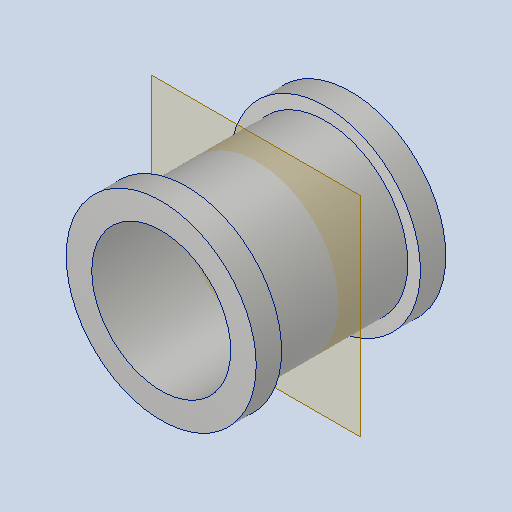
# Autodesk Inventor part: EL2-007
Saved by Autodesk Inventor 2023.4 (Build 274418000, 418)
## iProperties
Created: 2025-01-11
Part Number: EL2-007
Material: Aluminum 6061
Document SubType Name: Modeling
Designer: mavericks
Density: 2.7 g/cm^3
Appearance: Aluminum - Flat
Author: mavericks
Autodesk Inventor part; units mm, degrees
ref_plane "YZ Plane" through (0, 0, 0) normal (1, 0, 0) x (0, 1, 0)
ref_plane "XZ Plane" through (0, 0, 0) normal (0, 1, 0) x (-1, 0, 0)
sketch "Sketch1" plane through (0, 0, 0) normal (0, 0, 1) x (1, 0, 0)
  line L0 (-12.7, 76.2) -> (12.7, 76.2) construction
  line L1 (12.7, 76.2) -> (12.7, -76.2) construction
  line L2 (12.7, -76.2) -> (-12.7, -76.2) construction
  line L3 (-12.7, -76.2) -> (-12.7, 76.2) construction
  line L4 (-12.7, 76.2) -> (12.7, -76.2) construction
  line L5 (12.7, 76.2) -> (-12.7, -76.2) construction
  line L6 (19.05, 76.2) -> (44.45, 76.2) construction
  line L7 (44.45, 76.2) -> (44.45, -76.2) construction
  line L8 (44.45, -76.2) -> (19.05, -76.2) construction
  line L9 (19.05, -76.2) -> (19.05, 76.2) construction
  line L10 (19.05, 76.2) -> (44.45, -76.2) construction
  line L11 (44.45, 76.2) -> (19.05, -76.2) construction
  circle A0 centre (2.7686, 0) radius 8.6995
  line L12 (11.1125, -57.0186) -> (11.1125, 57.0186) construction
  line L13 (11.1125, 57.0186) -> (-14.2875, -95.3814) construction
  line L14 (-14.2875, -95.3814) -> (-14.2875, 95.3814) construction
  line L15 (-14.2875, 95.3814) -> (11.1125, -57.0186) construction
  line L16 (13.081, 27.2802) -> (13.081, -0.0011) construction
  circle A1 centre (2.7686, 0) radius 10.3124
  point P0 (0, 0)
  point P1 (31.75, 0)
  point P2 (0, 0)
  point P3 (0, 76.2)
  point P4 (31.75, 76.2)
  point P5 (0, 0)
  dimension "d1" = 25.4
  dimension "d2" = 152.4
  dimension "d3" = 25.4
  dimension "d4" = 152.4
  dimension "d5" = 6.35
  dimension "d6" = 17.399
  dimension "d7" = 1.5875
  dimension "d8" = 0.381
  dimension "d11" = 20.6248
  dimension "d21" = 9.9314
  constraints: 34 end point, 6 midpoint, 5 parallel, 2 centre point, 2 coincident, 2 horizontal, 2 horizontal alignment, 2 perpendicular, 1 tangent, 1 vertical, 3 other
  measures "d1" distance of L1.end L2.end
  measures "d2" distance of L0.end L1.end
  measures "d3" distance of L7.end L8.end
  measures "d4" distance of L6.end L7.end
  measures "d5" distance between parallel lines of L9 L1
  measures "d6" diameter of A0
  measures "d7" distance between parallel lines of L1 L12
  measures "d8" distance between parallel lines of L1 L16
  measures "d11" diameter of A1
  measures "d21" distance from line of A0.centre L1
extrude "Extrusion1" add sketch "Sketch1" along normal mid plane 17.399
sketch "Sketch2" plane through (2.7686, 0, 8.6995) normal (0, 0, 1) x (1, 0, 0)
  circle A0 centre (0, 0) radius 10.3124 projected
  circle A1 centre (0, 0) radius 11.8999
  circle A2 centre (0, 0) radius 8.6995 projected
  point P0 (-2.7686, 0)
  dimension "d14" = 1.5875
  constraints: 1 centre point
  measures "d14" radial gap between concentric circles of A0 A1
extrude "Extrusion2" add sketch "Sketch2" along normal blind 3.175 contours A0 | A1
sketch "Sketch3" plane through (2.7686, 0, -8.6995) normal (0, 0, -1) x (-1, 0, 0)
  circle A0 centre (0, 0) radius 10.3124 projected
  circle A1 centre (0, 0) radius 11.8999
  circle A2 centre (0, 0) radius 8.6995 projected
  point P0 (2.7686, 0)
  dimension "d17" = 1.5875
  dimension "d22" = 23.7998
  constraints: 1 centre point
  measures "d17" radial gap between concentric circles of A0 A1
  measures "d22" diameter of A1
extrude "Extrusion3" add sketch "Sketch3" along normal blind 3.175 contours A0 | A1
equation "\"d12\" = d6"
body "Solid1"
